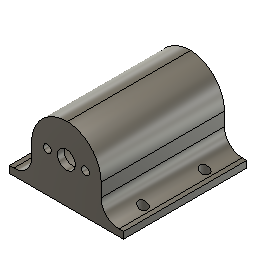
suporte-motor-encoder (Autodesk Fusion 360 design; units mm, degrees)
Autodesk Fusion 360 part; units mm, degrees
sketch "Sketch1" plane through (0, 0, 0) normal (0, 0, 1) x (1, 0, 0)
  line L0 (0, 0) -> (51, 0)
  line L1 (51, 0) -> (51, 33)
  line L2 (51, 33) -> (0, 33)
  line L3 (0, 33) -> (0, 0)
  dimension "d1" = 33
  dimension "d2" = 51
  constraint coincident L0.start L3.end
  constraint horizontal L0
  constraint perpendicular L0 L1
  constraint perpendicular L1 L2
  constraint perpendicular L2 L3
  measures "d1" distance of L0.end L1.end
  measures "d2" distance of L1.end L2.end
extrude "Extrude1" add sketch "Sketch1" along normal blind 55
sketch "Sketch2" plane through (0, 0, 55) normal (0, 0, 1) x (1, 0, 0)
  line L0 (0, 33) -> (0, 0)
  line L1 (0, 0) -> (51, 0)
  line L2 (51, 0) -> (51, 33)
  line L3 (51, 33) -> (0, 33)
  line L4 (0, 3) -> (10, 3)
  line L5 (10, 3) -> (10, 33)
  line L6 (41, 33) -> (41, 3)
  line L7 (41, 3) -> (51, 3)
  dimension "d5" = 10
  dimension "d6" = 10
  dimension "d7" = 3
  dimension "d8" = 3
  constraint coincident L0 L4.start
  constraint perpendicular L0 L4
  constraint coincident L3 L5.end
  constraint perpendicular L3 L5
  constraint coincident L3 L6.start
  constraint perpendicular L3 L6
  constraint coincident L2 L7.end
  constraint perpendicular L2 L7
  measures "d5" distance of L4.start L4.end
  measures "d6" distance of L6.end L7.end
  measures "d7" distance of L1.end L7.end
  measures "d8" distance of L0.end L4.start
extrude "Extrude2" cut sketch "Sketch2" against normal blind 55 contours L0 L3 L4 L5 | L2 L3 L6 L7
sketch "Sketch3" plane through (0, 0, 0) normal (0, 0, -1) x (-1, 0, 0)
  line L0 (-10, 3) -> (-10, 33)
  line L1 (-10, 33) -> (-41, 33)
  line L2 (-41, 33) -> (-41, 3)
  line L3 (-41, 3) -> (-51, 3)
  line L4 (-51, 3) -> (-51, 0)
  line L5 (-51, 0) -> (0, 0)
  line L6 (0, 0) -> (0, 3)
  line L7 (0, 3) -> (-10, 3)
  line L8 (-25.5, 33) -> (-25.5, 0) construction
  line L9 (-41, 18) -> (-10, 18) construction
  circle A0 centre (-25.5, 18) radius 12.5
  dimension "d11" = 25
  constraint midpoint L1 L8.start
  constraint midpoint L5 L8.end
  constraint midpoint L2 L9.start
  constraint midpoint L0 L9.end
  constraint midpoint L9 A0.centre
  measures "d11" diameter of A0
extrude "Extrude3" cut sketch "Sketch3" against normal blind 52 contours A0
sketch "Sketch4" plane through (0, 0, 52) normal (0, 0, -1) x (-1, 0, 0)
  circle A0 centre (-25.5, 18) radius 12.5
  circle A1 centre (-25.5, 18) radius 4
  dimension "d14" = 8
  constraint concentric A0 A1
  measures "d14" diameter of A1
extrude "Extrude4" cut sketch "Sketch4" against normal blind 3 contours A1
sketch "Sketch5" plane through (0, 0, 55) normal (0, 0, 1) x (1, 0, 0)
  circle A0 centre (25.5, 18) radius 4
  line L0 (10, 3) -> (0, 3)
  line L1 (0, 3) -> (0, 0)
  line L2 (0, 0) -> (51, 0)
  line L3 (51, 0) -> (51, 3)
  line L4 (51, 3) -> (41, 3)
  line L5 (41, 3) -> (41, 33)
  line L6 (41, 33) -> (10, 33)
  line L7 (10, 33) -> (10, 3)
  circle A1 centre (25.5, 18) radius 13.5 construction
  line L8 (10, 18) -> (41, 18) construction
  circle A2 centre (17, 18) radius 1.75
  circle A3 centre (34, 18) radius 1.75
  dimension "d17" = 27
  dimension "d18" = 3.5
  dimension "d19" = 3.5
  dimension "d20" = 8.5
  dimension "d21" = 8.5
  constraint concentric A0 A1
  constraint midpoint L7 L8.start
  constraint midpoint L5 L8.end
  constraint coincident L8 A2.centre
  constraint coincident L8 A3.centre
  measures "d17" diameter of A1
  measures "d18" diameter of A2
  measures "d19" diameter of A3
  measures "d20" distance of A0.centre A2.centre
  measures "d21" distance of A0.centre A3.centre
extrude "Extrude5" cut sketch "Sketch5" against normal blind 3 contours A2 | A3
fillet "Fillet1" radius 16 2 edges at (10, 33, 27.5) (41, 33, 27.5)
fillet "Fillet2" radius 8 2 edges at (41, 3, 27.5) (10, 3, 27.5)
sketch "Sketch6" plane through (0, 0, 0) normal (0, -1, 0) x (1, 0, 0)
  line L0 (0, 0) -> (51, 0)
  line L1 (51, 0) -> (51, 55)
  line L2 (51, 55) -> (0, 55)
  line L3 (0, 55) -> (0, 0)
  line L4 (5, 55) -> (5, 0) construction
  line L5 (46, 55) -> (46, 0) construction
  line L6 (0, 41.25) -> (51, 41.25) construction
  line L7 (0, 13.75) -> (51, 13.75) construction
  circle A0 centre (5, 13.75) radius 2
  circle A1 centre (46, 13.75) radius 2
  circle A2 centre (5, 41.25) radius 2
  circle A3 centre (46, 41.25) radius 2
  dimension "d26" = 5
  dimension "d27" = 5
  dimension "d28" = 13.75
  dimension "d29" = 13.75
  dimension "d30" = 4
  dimension "d31" = 4
  dimension "d32" = 4
  dimension "d33" = 4
  constraint coincident L2 L4.start
  constraint coincident L0 L4.end
  constraint perpendicular L0 L4
  constraint coincident L2 L5.start
  constraint coincident L0 L5.end
  constraint perpendicular L0 L5
  constraint coincident L3 L6.start
  constraint coincident L1 L6.end
  constraint perpendicular L1 L6
  constraint coincident L3 L7.start
  constraint coincident L1 L7.end
  constraint perpendicular L1 L7
  constraint coincident L7 A0.centre
  constraint coincident L4 A0.centre
  constraint coincident L7 A1.centre
  constraint coincident L5 A1.centre
  constraint coincident L6 A2.centre
  constraint coincident L4 A2.centre
  constraint coincident L5 A3.centre
  constraint coincident L6 A3.centre
  measures "d26" distance of L3 L4
  measures "d27" distance of L1 L5
  measures "d28" distance of L0 L7
  measures "d29" distance of L2 L6
  measures "d30" diameter of A0
  measures "d31" diameter of A1
  measures "d32" diameter of A2
  measures "d33" diameter of A3
extrude "Extrude6" cut sketch "Sketch6" against normal blind 5 contours A0 | A1 | A2 | A3
sketch "Sketch7" plane through (0, 0, 0) normal (0, 0, -1) x (-1, 0, 0)
  circle A0 centre (-25.5, 18) radius 12.5
  arc A1 (-26, 33) -> (-41, 17.0313) centre (-25, 17.0313) ccw
  line L0 (-41, 17.0313) -> (-41, 11)
  arc A2 (-49, 3) -> (-41, 11) centre (-49, 11) ccw
  line L1 (-49, 3) -> (-51, 3)
  line L2 (-51, 3) -> (-51, 0)
  line L3 (-51, 0) -> (0, 0)
  line L4 (0, 0) -> (0, 3)
  line L5 (0, 3) -> (-2, 3)
  arc A3 (-10, 11) -> (-2, 3) centre (-2, 11) ccw
  line L6 (-10, 11) -> (-10, 17)
  arc A4 (-10, 17) -> (-26, 33) centre (-26, 17) ccw
  line L7 (-25.5, 18) -> (-21.5, 18)
  circle A5 centre (-25.5, 18) radius 13.5
  dimension "d36" = 27
  constraint coincident A0.centre L7.start
  constraint horizontal L7
  measures "d36" diameter of A5
extrude "Extrude7" cut sketch "Sketch7" against normal blind 52 contours A5
